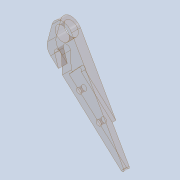
# Autodesk Inventor part: アーム先端
Saved by Autodesk Inventor 2020.4 (Build 244396000, 396)
## iProperties
Created: 2021-05-06
Part Number: アーム先端
Material: ポリカーボネート、スモーク
Document SubType Name: Modeling
Designer: happy
Density: 1.2 g/cm^3
Appearance: ポリカーボネート - スモーク
Mass: 3.25315 g
Surface Area: 22.7173 cm^2
Volume: 2.71096 cm^3
Author: happy
Autodesk Inventor part; units mm, degrees
ref_plane "YZ Plane" through (0, 0, 0) normal (1, 0, 0) x (0, 1, 0)
ref_plane "XZ Plane" through (0, 0, 0) normal (0, 1, 0) x (-1, 0, 0)
ref_plane "XY Plane" through (0, 0, 0) normal (0, 0, 1) x (1, 0, 0)
sketch "スケッチ1" plane through (0, 0, 0) normal (0, 0, 1) x (1, 0, 0)
  circle A0 centre (295.848871, -93.120076) radius 1.5
  circle A1 centre (295.848871, -93.120076) radius 3.025
  line L0 (302.911618, -92.777137) -> (291.344796, -101.566309)
  arc A2 (282.40584, -101.176779) -> (291.344796, -101.566309) centre (287.109706, -95.992799) ccw
  arc A3 (299.078829, -95.689522) -> (299.346701, -89.542385) centre (296.658778, -92.504659) ccw
  line L1 (214.413679, -12.475426) -> (302.911618, -92.777137)
  line L2 (186.870748, -14.489658) -> (289.472001, -107.588508)
  line L3 (89.513673, -53) -> (377.048162, -53)
  circle A4 centre (295.848871, -93.120076) radius 4.025
  circle A5 centre (295.848871, -93.120076) radius 6
  line L4 (290.052231, -91.571215) -> (285.593636, -108.257588)
  circle A6 centre (285.42622, -97.165857) radius 3.025
  arc A7 (287.438666, -101.35253) -> (289.20342, -107.344802) centre (293.235305, -102.901391) ccw
  circle A8 centre (298.015884, -108.589531) radius 3
  circle A9 centre (298.015884, -108.589531) radius 1.5
  line L5 (185.106531, 0.614305) -> (481.333939, -268.178035)
  line L6 (295.848871, -93.120076) -> (289.20342, -100.443813) construction
  line L7 (301.069617, -90.163082) -> (333.637532, -147.663653)
  line L8 (333.637532, -147.663653) -> (289.20342, -107.344802)
  circle A10 centre (295.848871, -93.120076) radius 1.5
  circle A11 centre (295.848871, -93.120076) radius 3.025
  line L9 (302.911618, -92.777137) -> (291.344796, -101.566309)
  arc A12 (282.40584, -101.176779) -> (291.344796, -101.566309) centre (287.109706, -95.992799) ccw
  arc A13 (299.078829, -95.689522) -> (299.346701, -89.542385) centre (296.658778, -92.504659) ccw
  line L10 (214.413679, -12.475426) -> (302.911618, -92.777137)
  line L11 (186.870748, -14.489658) -> (289.472001, -107.588508)
  line L12 (89.513673, -53) -> (377.048162, -53)
  circle A14 centre (295.848871, -93.120076) radius 4.025
  circle A15 centre (295.848871, -93.120076) radius 6
  line L13 (290.052231, -91.571215) -> (285.593636, -108.257588)
  circle A16 centre (285.42622, -97.165857) radius 3.025
  arc A17 (287.438666, -101.35253) -> (289.20342, -107.344802) centre (293.235305, -102.901391) ccw
  circle A18 centre (298.015884, -108.589531) radius 3 construction
  circle A19 centre (298.015884, -108.589531) radius 1.5
  line L14 (185.106531, 0.614305) -> (481.333939, -268.178035)
  line L15 (295.848871, -93.120076) -> (289.20342, -100.443813) construction
  line L16 (301.069617, -90.163082) -> (333.637532, -147.663653)
  line L17 (333.637532, -147.663653) -> (289.20342, -107.344802)
  line L18 (301.984952, -108.140062) -> (343.184474, -145.523895)
  circle A20 centre (305.221577, -116.478183) radius 1.5
  circle A21 centre (316.330105, -126.557896) radius 1.5
  line L19 (301.984952, -108.140062) -> (293.498432, -117.492783)
  arc A22 (303.540146, -109.551222) -> (301.984952, -108.140062) centre (302.762549, -108.845642) ccw
  line L20 (301.984952, -108.140062) -> (302.762549, -108.845642) construction
  line L21 (303.540146, -109.551222) -> (302.762549, -108.845642) construction
  point P0 (0, 0)
  point P1 (0, 0)
  point P2 (297.912288, -96.575931)
  point P3 (298.625557, -96.033946)
  point P4 (0, 0)
  point P5 (296.609105, -114.064611)
  point P6 (321.049741, -125.439168)
  dimension "d0" = 8.05
  dimension "d1" = 12
  dimension "d2" = 6
  dimension "d3" = 6
  dimension "d4" = 3
  dimension "d5" = 5
  dimension "d6" = 12
  dimension "d7" = 60
  dimension "d11" = 8.05
  dimension "d12" = 12
  dimension "d13" = 6
  dimension "d14" = 6
  dimension "d15" = 3
  dimension "d16" = 5
  dimension "d17" = 12
  dimension "d18" = 60
  dimension "d19" = 8
  dimension "d20" = 4
  dimension "d21" = 4
  dimension "d22" = 3
  dimension "d23" = 50
  dimension "d24" = 8
  dimension "d25" = 15
  dimension "d28" = 1.05
  dimension "d29" = 180
  constraints: 44 end point, 23 centre point, 18 point on circle, 13 tangent, 6 coincident, 6 point on line, 3 perpendicular, 1 equal radius, 12 other
  measures "d0" diameter of A4
  measures "d1" diameter of A5
  measures "d2" radius of A7
  measures "d3" diameter of A8
  measures "d4" diameter of A9
  measures "d5" distance from line of A9.centre L5
  measures "d6" distance from line of A8.centre L6
  measures "d7" distance of L7.end L8.end
  measures "d11" diameter of A14
  measures "d12" diameter of A15
  measures "d13" radius of A17
  measures "d14" diameter of A18
  measures "d15" diameter of A19
  measures "d16" distance from line of A19.centre L14
  measures "d17" distance from line of A18.centre L15
  measures "d18" distance of L16.end L17.end
  measures "d19" distance between parallel lines of L17 L18
  measures "d20" distance from line of L18 A20.centre
  measures "d21" distance from line of L18 A21.centre
  measures "d22" diameter of A20
  measures "d23" distance from line of L16.end L19
  measures "d24" distance from line of L19 A20.centre
  measures "d25" distance between centres of A21 A20
  measures "d28" radius of A22
  measures "d29" angle of L20 L21
extrude "押し出し1" add sketch "スケッチ1" along normal blind 5 contours L7 L5 A5 L0 | L0 A5 L1 L7 | L1 A5 L7 | A5 L5 L0 A4 | L0 A3 L1 A5 | L7 L18 A22 L19 A8 L8 L2 A7 A2 L0 A5 L5 | L1 A5 | L0 A4 L5 A5 L1 A3 | A5 L0 L5 | L7 L8 L19 A8 L18 | A4 L0 | A5 L5 L0 | L0 A2 A7 L4 L5 A5 | L18 A22 | A5 L5 L4 | L19 A8 | A8 L19 | A9 picked at (298.233704, -96.341002)
fillet "フィレット1" radius 1 1 edges at (333.6375, -147.6637, 2.5)
extrude "押し出し2" cut sketch "スケッチ1" along normal blind 2 contours L7 L8 L19 A8 L18 | L18 A22 | L19 A8 picked at (299.870596, -110.60445)
sketch "スケッチ2" plane through (0, 0, 5) normal (0, 0, 1) x (1, 0, 0)
  arc A0 (329.027651, -143.480716) -> (330.569756, -142.247316) centre (329.699632, -142.740148) ccw
  line L0 (330.569756, -142.247316) -> (301.069617, -90.163082)
  arc A1 (301.069617, -90.163082) -> (290.052231, -91.571215) centre (295.848871, -93.120076) ccw
  line L1 (290.052231, -91.571215) -> (287.438666, -101.35253)
  arc A2 (287.438666, -101.35253) -> (289.20342, -107.344802) centre (293.235305, -102.901391) ccw
  line L2 (289.20342, -107.344802) -> (329.027651, -143.480716)
  arc A3 (298.625557, -96.033946) -> (297.912288, -96.575931) centre (295.848871, -93.120076) ccw
  line L3 (298.625557, -96.033946) -> (297.912288, -96.575931)
  circle A4 centre (316.330105, -126.557896) radius 1.5
  circle A5 centre (305.221577, -116.478183) radius 1.5
  line L4 (301.984952, -108.140062) -> (296.609105, -114.064611)
  line L5 (289.20342, -107.344802) -> (296.609105, -114.064611)
  line L6 (293.646831, -111.376687) -> (291.510724, -104.715452)
  line L7 (295.412844, -104.007733) -> (295.868537, -113.39263)
  arc A6 (295.412844, -104.007733) -> (291.510724, -104.715452) centre (293.415198, -104.104731) ccw
  point P0 (0, 0)
  point P1 (293.646831, -111.376687)
  dimension "d31" = 30
  dimension "d32" = 45
  dimension "d33" = 3
  dimension "d34" = 2
  dimension "d37" = 1
  constraints: 4 end point, 2 point on circle, 2 point on line, 2 tangent, 1 centre point
  measures "d31" angle of L5 L6
  measures "d32" angle of L5 L7
  measures "d33" distance of L7.end L6.start
  measures "d34" radius of A6
  measures "d37" distance from line of L4 L7.end
extrude "押し出し3" cut sketch "スケッチ2" against normal blind 10 contours L2 L6 A6 L7
equation "\"d20\" = 0.5 * d19"
equation "\"d21\" = d20"
